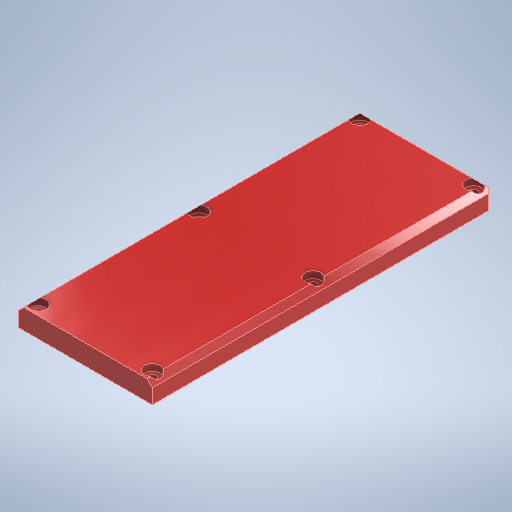
# Autodesk Inventor part: Top Covers
Saved by Autodesk Inventor 2026.2 (Build 302298010, 298A)
## iProperties
Created: 2026-05-07
Part Number: Top Covers
Material: Generic
Document SubType Name: Modeling
Designer: piete
Density: 1 g/cm^3
Appearance: Orange-Red
Author: piete
Autodesk Inventor part; units mm, degrees
ref_plane "YZ Plane" through (0, 0, 0) normal (1, 0, 0) x (0, 1, 0)
ref_plane "XZ Plane" through (0, 0, 0) normal (0, 1, 0) x (-1, 0, 0)
ref_plane "XY Plane" through (0, 0, 0) normal (0, 0, 1) x (1, 0, 0)
sketch "Sketch1" plane through (0, 0, 0) normal (0, 1, 0) x (-1, 0, 0)
  line L0 (25, 63.75) -> (-25, 63.75)
  line L1 (-25, 63.75) -> (-25, -63.75)
  line L2 (-25, -63.75) -> (25, -63.75)
  line L3 (25, -63.75) -> (25, 63.75)
  point P0 (0, 0)
  dimension "d0" = 50
  dimension "d1" = 127.5
  dimension "d2" = 25
  dimension "d3" = 63.75
  constraints: 8 end point, 2 parallel, 1 horizontal, 1 perpendicular
  measures "d0" distance of L2.end L1.end
  measures "d1" distance of L1.end L0.end
  measures "d2" distance from line of point (0, 0) L3
  measures "d3" distance from line of point (0, 0) L0
extrude "Extrusion1" add sketch "Sketch1" along normal blind 7.5
sketch "Sketch2" plane through (0, 7.5, 0) normal (0, 1, 0) x (1, 0, 0)
  circle A0 centre (-21.25, -60) radius 1.5
  circle A1 centre (-21.25, 60) radius 1.5
  circle A2 centre (21.25, -60) radius 1.5
  circle A3 centre (21.25, 60) radius 1.5
  circle A4 centre (-21.25, 0) radius 1.5
  circle A5 centre (21.25, 0) radius 1.5
  line L0 (25, -63.75) -> (25, 63.75) projected
  line L1 (25, 63.75) -> (-25, 63.75) projected
  line L2 (-25, -63.75) -> (25, -63.75) projected
  line L3 (-25, 63.75) -> (-25, -63.75) projected
  point P0 (0, 0)
  dimension "d6" = 3
  dimension "d7" = 3
  dimension "d8" = 3
  dimension "d9" = 3
  dimension "d10" = 3
  dimension "d11" = 3
  dimension "d12" = 3.75
  dimension "d13" = 3.75
  dimension "d14" = 3.75
  dimension "d15" = 3.75
  dimension "d16" = 3.75
  dimension "d17" = 3.75
  dimension "d18" = 3.75
  dimension "d19" = 3.75
  dimension "d20" = 3.75
  dimension "d21" = 3.75
  dimension "d22" = 63.75
  dimension "d23" = 63.75
  constraints: 6 centre point
  measures "d6" diameter of A0
  measures "d7" diameter of A1
  measures "d8" diameter of A2
  measures "d9" diameter of A3
  measures "d10" diameter of A4
  measures "d11" diameter of A5
  measures "d12" distance from line of L0 A5.centre
  measures "d13" distance from line of L0 A3.centre
  measures "d14" distance from line of L1 A3.centre
  measures "d15" distance from line of L0 A2.centre
  measures "d16" distance from line of L2 A2.centre
  measures "d17" distance from line of L3 A0.centre
  measures "d18" distance from line of L2 A0.centre
  measures "d19" distance from line of L3 A4.centre
  measures "d20" distance from line of L1 A1.centre
  measures "d21" distance from line of L3 A1.centre
  measures "d22" distance from line of L1 A4.centre
  measures "d23" distance from line of L1 A5.centre
extrude "Extrusion2" cut sketch "Sketch2" against normal through all contours A0 | A1 | A2 | A3 | A4 | A5
sketch "Sketch3" plane through (0, 7.5, 0) normal (0, 1, 0) x (1, 0, 0)
  circle A0 centre (21.25, -60) radius 1.5 projected
  circle A1 centre (21.25, -60) radius 3
  circle A2 centre (21.25, 0) radius 1.5 projected
  circle A3 centre (21.25, 0) radius 3
  circle A4 centre (21.25, 60) radius 3
  line L0 (25, 63.75) -> (-25, 63.75) projected
  line L1 (25, -63.75) -> (25, 63.75) projected
  point P0 (0, 0)
  dimension "d26" = 6
  dimension "d27" = 6
  dimension "d28" = 6
  dimension "d29" = 3.75
  dimension "d30" = 3.75
  constraints: 3 centre point, 2 coincident
  measures "d26" diameter of A1
  measures "d27" diameter of A3
  measures "d28" diameter of A4
  measures "d29" distance from line of L0 A4.centre
  measures "d30" distance from line of L1 A4.centre
extrude "Extrusion3" cut sketch "Sketch3" against normal blind 2.5
mirror "Mirror1" about plane through (0, 0, 0) normal (1, 0, 0) of "Extrusion3"
chamfer "Chamfer1" distance 2 angle 45 3 edges at (25, 7.5, 0) (0, 7.5, -63.75) (-25, 7.5, 0)
chamfer "Chamfer2" distance 2 angle 45 2 edges at (-25, 2.75, -63.75) (25, 2.75, -63.75)
equation "\"d2\" = 0.5 * d0"
equation "\"d3\" = 0.5 * d1"
equation "\"d12\" = 0.5 * Thickness"
equation "\"d13\" = 0.5 * Thickness"
equation "\"d14\" = 0.5 * Thickness"
equation "\"d15\" = 0.5 * Thickness"
equation "\"d16\" = 0.5 * Thickness"
equation "\"d17\" = 0.5 * Thickness"
equation "\"d18\" = 0.5 * Thickness"
equation "\"d19\" = 0.5 * Thickness"
equation "\"d20\" = 0.5 * Thickness"
equation "\"d21\" = 0.5 * Thickness"
equation "\"d22\" = 0.5 * d1"
equation "\"d23\" = 0.5 * d1"
equation "\"d29\" = 0.5 * Thickness"
equation "\"d30\" = 0.5 * Thickness"
equation "\"Thickness\" = 7.5"
body "Solid1"
